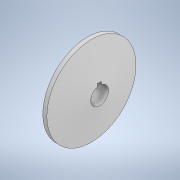
# Autodesk Inventor part: Nivelador de Correia
Saved by Autodesk Inventor 2022.1 (Build 261234020, 234B)
## iProperties
Created: 2023-08-25
Part Number: Nivelador de Correia
Material: Generic
Document SubType Name: Modeling
Designer: SENAI
Density: 1 g/cm^3
Appearance: Default
Author: SENAI
Autodesk Inventor part; units mm, degrees
ref_plane "YZ Plane" through (0, 0, 0) normal (1, 0, 0) x (0, 1, 0)
ref_plane "XZ Plane" through (0, 0, 0) normal (0, 1, 0) x (-1, 0, 0)
ref_plane "XY Plane" through (0, 0, 0) normal (0, 0, 1) x (1, 0, 0)
sketch "Sketch1" plane through (0, 0, 0) normal (0, 0, 1) x (1, 0, 0)
  line L0 (0, 87.5) -> (8, 87.5)
  line L1 (24, 0) -> (24, 17.5)
  line L2 (8, 87.5) -> (24, 17.5)
  line L3 (16, 0) -> (16, 17.5)
  line L4 (16, 17.5) -> (0, 87.5)
  line L5 (16, 0) -> (24, 0)
  point P0 (0, 0)
  dimension "d0" = 87.5
  dimension "d1" = 8
  dimension "d3" = 17.5
  dimension "d7" = 8
  dimension "d8" = 167.125
  dimension "d9" = 175
  dimension "d10" = 24
  constraints: 12 end point, 2 parallel, 2 vertical, 1 horizontal
  measures "d0" distance of point (0, 0) L0.start
  measures "d1" distance of L0.start L0.end
  measures "d3" distance of L1.start L1.end
  measures "d7" distance of L1.start L3.start
  measures "d8" angle of L1 L2
  measures "d9" diameter of L0 L5
  measures "d10" distance from line of point (0, 0) L1
revolve "Revolution1" add sketch "Sketch1" angle 360 about axis through (16, 0, 0) along (1, 0, 0)
sketch "Sketch2" plane through (0, 0, 0) normal (0, 0, 1) x (1, 0, 0)
  line L0 (16, 0) -> (16, 24.5)
  line L1 (16, -17.5) -> (16, 17.5) projected
  line L2 (14.4, 24.5) -> (16, 24.5)
  line L3 (14.4, 24.5) -> (-13.6, 24.5)
  line L4 (-13.6, 24.5) -> (-13.6, 0)
  line L5 (-13.6, 0) -> (16, 0)
  point P0 (0, 0)
  dimension "d13" = 24.5
  dimension "d15" = 28
  constraints: 10 end point, 2 horizontal, 1 collinear, 1 vertical
  measures "d13" distance of L0.start L0.end
  measures "d15" distance of L2.start L3.end
revolve "Revolution2" add sketch "Sketch2" angle 360 about axis through (-13.6, 0, 0) along (1, 0, 0)
sketch "Sketch3" plane through (0, 0, 0) normal (0, 0, 1) x (1, 0, 0)
  line L0 (14.4, 0) -> (14.4, 30.5)
  line L1 (14.4, 30.5) -> (13.0159, 30.5)
  line L2 (13.0159, 30.5) -> (9.0159, 30.5)
  line L3 (9.0159, 30.5) -> (9.0159, 0)
  line L4 (9.0159, 0) -> (14.4, 0)
  point P0 (0, 0)
  dimension "d17" = 30.5
  dimension "d18" = 4
  constraints: 10 end point, 2 horizontal, 1 point on line, 1 vertical
  measures "d17" distance of L0.start L0.end
  measures "d18" distance of L1.end L2.end
revolve "Revolution3" add sketch "Sketch3" angle 360 about axis through (9.0159, 0, 0) along (1, 0, 0)
sketch "Sketch4" plane through (24, 0, 0) normal (1, 0, 0) x (0, 0, -1)
  circle A0 centre (0, 0) radius 17.5
  constraints: 1 centre point, 1 coincident
extrude "Extrusion1" cut sketch "Sketch4" against normal through all
sketch "Sketch5" plane through (-13.6, 0, 0) normal (-1, 0, 0) x (0, 0, 1)
  circle A0 centre (0, 0) radius 17.5 projected
  line L0 (0, 21.5) -> (4, 21.5)
  line L1 (0, 21.5) -> (-4, 21.5)
  line L2 (-4, 21.5) -> (-4, 17.0367)
  line L3 (4, 21.5) -> (4, 17.0367)
  line L4 (-4, 17.0367) -> (4, 17.0367)
  dimension "d23" = 4
  dimension "d24" = 4
  constraints: 10 end point, 3 point on circle, 2 horizontal, 2 vertical
  measures "d23" distance of L0.start L0.end
  measures "d24" distance of L0.start L1.end
extrude "Extrusion2" cut sketch "Sketch5" against normal through all contours A0 L2 L1 L0 L3
body "Solid1"
